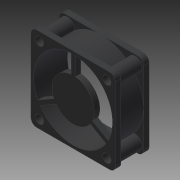
# Autodesk Inventor part: Cooler
Saved by Autodesk Inventor 2014 SP1 (Build 180222100, 222)
## iProperties
Created: 2017-12-02
Part Number: Cooler
Material: Типовые
Document SubType Name: Modeling
Designer: Stepan
Density: 1 g/cm^3
Appearance: Типовые
Author: Stepan
Autodesk Inventor part; units mm, degrees
ref_plane "YZ Plane" through (0, 0, 0) normal (1, 0, 0) x (0, 1, 0)
ref_plane "XZ Plane" through (0, 0, 0) normal (0, 1, 0) x (-1, 0, 0)
ref_plane "XY Plane" through (0, 0, 0) normal (0, 0, 1) x (1, 0, 0)
sketch "Эскиз1" plane through (0, 0, 0) normal (0, 1, 0) x (-1, 0, 0)
  line L0 (-12, 12) -> (12, 12) construction
  line L1 (12, 12) -> (12, -12) construction
  line L2 (12, -12) -> (-12, -12) construction
  line L3 (-12, -12) -> (-12, 12) construction
  line L4 (-12, 12) -> (12, -12) construction
  line L5 (12, 12) -> (-12, -12) construction
  line L6 (-15, -15) -> (15, -15)
  line L7 (15, -15) -> (15, 15)
  line L8 (15, 15) -> (-15, 15)
  line L9 (-15, 15) -> (-15, -15)
  line L10 (-15, -15) -> (15, 15) construction
  line L11 (15, -15) -> (-15, 15) construction
  circle A0 centre (0, 0) radius 14
  circle A1 centre (-12, -12) radius 1.5
  circle A2 centre (-12, 12) radius 1.5
  circle A3 centre (12, 12) radius 1.5
  circle A4 centre (12, -12) radius 1.5
  dimension "d0" = 24
  dimension "d1" = 24
  dimension "d2" = 30
  dimension "d3" = 30
  dimension "d4" = 28
  dimension "d8" = 3
  dimension "d9" = 3
  dimension "d10" = 3
  dimension "d11" = 3
  constraints: 24 end point, 5 centre point, 4 coincident, 4 midpoint, 4 parallel, 2 horizontal, 2 perpendicular, 2 point on line
  measures "d0" distance of L1.end L2.end
  measures "d1" distance of L0.end L1.end
  measures "d2" distance of L8.end L7.end
  measures "d3" distance of L7.end L6.end
  measures "d4" diameter of A0
  measures "d8" diameter of A1
  measures "d9" diameter of A2
  measures "d10" diameter of A3
  measures "d11" diameter of A4
extrude "Выдавливание1" add sketch "Эскиз1" along normal blind 2
sketch "Эскиз2" plane through (0, 0, 0) normal (0, -1, 0) x (1, 0, 0)
  circle A0 centre (0, 0) radius 14 projected
  circle A1 centre (-12, -12) radius 1.5 projected
  circle A2 centre (-12, 12) radius 1.5 projected
  circle A3 centre (12, 12) radius 1.5 projected
  circle A4 centre (12, -12) radius 1.5 projected
  circle A5 centre (0, 0) radius 15
  circle A6 centre (-12, -12) radius 2.5
  circle A7 centre (-12, 12) radius 2.5
  circle A8 centre (12, 12) radius 2.5
  circle A9 centre (12, -12) radius 2.5
  dimension "d14" = 5
  dimension "d15" = 5
  dimension "d16" = 5
  dimension "d17" = 5
  constraints: 5 centre point, 5 coincident
  measures "d14" diameter of A6
  measures "d15" diameter of A7
  measures "d16" diameter of A8
  measures "d17" diameter of A9
extrude "Выдавливание2" add sketch "Эскиз2" along normal blind 8
sketch "Эскиз4" plane through (0, -8, 0) normal (0, -1, 0) x (1, 0, 0)
  circle A0 centre (12, 12) radius 1.5 projected
  circle A1 centre (-12, -12) radius 1.5 projected
  circle A2 centre (-12, 12) radius 1.5 projected
  circle A3 centre (12, -12) radius 1.5 projected
  circle A4 centre (0, 0) radius 14 projected
  arc A5 (11.5789, -9.5357) -> (11.5789, 9.5357) centre (0, 0) ccw projected
  line L0 (-15, 15) -> (15, 15)
  line L1 (15, 15) -> (15, -15)
  line L2 (15, -15) -> (-15, -15)
  line L3 (-15, -15) -> (-15, 15)
  circle A6 centre (0, 0) radius 7.5
  line L4 (0, 0) -> (0, 15) construction
  line L5 (0, 0) -> (-12.1244, -7) construction
  line L6 (0, 0) -> (12.1244, -7) construction
  line L7 (-0.75, 6.7531) -> (0.75, 6.7531)
  line L8 (0.75, 6.7531) -> (0.75, 14.2469)
  line L9 (0.75, 14.2469) -> (-0.75, 14.2469)
  line L10 (-0.75, 14.2469) -> (-0.75, 6.7531)
  line L11 (-0.75, 6.7531) -> (0.75, 14.2469) construction
  line L12 (0.75, 6.7531) -> (-0.75, 14.2469) construction
  line L13 (-5.565, -4.079) -> (-6.315, -2.7799)
  line L14 (-6.315, -2.7799) -> (-12.8048, -6.5268)
  line L15 (-12.8048, -6.5268) -> (-12.0548, -7.8259)
  line L16 (-12.0548, -7.8259) -> (-5.565, -4.079)
  line L17 (-5.565, -4.079) -> (-12.8048, -6.5268) construction
  line L18 (-6.315, -2.7799) -> (-12.0548, -7.8259) construction
  line L19 (6.315, -2.7799) -> (5.565, -4.079)
  line L20 (5.565, -4.079) -> (12.0548, -7.8259)
  line L21 (12.0548, -7.8259) -> (12.8048, -6.5268)
  line L22 (12.8048, -6.5268) -> (6.315, -2.7799)
  line L23 (6.315, -2.7799) -> (12.0548, -7.8259) construction
  line L24 (5.565, -4.079) -> (12.8048, -6.5268) construction
  point P0 (0, 10.5)
  point P1 (-9.1849, -5.3029)
  point P2 (9.1849, -5.3029)
  dimension "d22" = 15
  dimension "d23" = 120
  dimension "d24" = 120
  dimension "d25" = 1.5
  dimension "d26" = 1.5
  dimension "d27" = 1.5
  constraints: 50 end point, 8 parallel, 7 midpoint, 4 perpendicular, 3 point on line, 2 horizontal, 2 point on circle, 1 centre point, 1 coincident
  measures "d22" diameter of A6
  measures "d23" angle of L5 L4
  measures "d24" angle of L6 L4
  measures "d25" distance of L9.end L8.end
  measures "d26" distance of L16.start L14.end
  measures "d27" distance of L22.start L20.end
extrude "Выдавливание4" add sketch "Эскиз4" along normal blind 2 contours L8 A6 L10 A4 | A4 L10 L9 L8 | L22 L21 L20 A4 | A4 L20 A6 L22 | L8 L7 L10 A6 | A6 L22 L19 L20 L16 L13 L14 L10 L7 L8 | A6 L20 L19 L22 | L14 A6 L16 A4 | A4 L16 L15 L14 | L14 L13 L16 A6 | L0 L1 L2 L3
fillet "Сопряжение1" radius 2 8 edges at (-15, -9, -15) (15, -9, -15) (15, 1, -15) (-15, 1, -15) (-15, 1, 15) (-15, -9, 15) (15, 1, 15) (15, -9, 15)
